Autodesk Fusion 360 part; units mm, degrees
(part 2 of 2)
sketch "Sketch10" plane through (25, 0, 0) normal (-1, 0, 0) x (0, -1, 0)
  arc A0 (-34, 37) -> (-40, 31) centre (-34, 31) ccw
  line L0 (-40, 31) -> (-40, 5)
  line L1 (-40, 5) -> (-10, 5)
  line L2 (-10, 5) -> (-10, 31)
  arc A1 (-10, 31) -> (-16, 37) centre (-16, 31) ccw
  line L3 (-16, 37) -> (-34, 37)
  arc A2 (-21.0078, 28.25) -> (-28.9922, 28.25) centre (-25, 28.5) ccw
  arc A3 (-21.0001, 28.0281) -> (-21.0078, 28.25) centre (-25, 28) ccw
  line L4 (-21.0001, 28.0281) -> (-22.5107, 11.7687)
  arc A4 (-27.4899, 11.7754) -> (-22.5107, 11.7687) centre (-25, 12) ccw
  line L5 (-27.4899, 11.7754) -> (-28.8938, 27.1715)
  line L6 (-28.8938, 27.1715) -> (-28.9999, 28.0281)
  arc A5 (-28.9922, 28.25) -> (-28.9999, 28.0281) centre (-25, 28) ccw
  circle A6 centre (-25, 28.5) radius 4
  circle A7 centre (-25, 12) radius 2.5
  line L7 (-22.5107, 11.7687) -> (-21.0001, 28.0281)
  line L8 (-28.9999, 28.0281) -> (-27.4899, 11.7754)
  constraint concentric A2 A6
  constraint concentric A4 A7
  constraint coincident L4.end A4.end
  constraint coincident A3.start L4.start
  constraint coincident L6.end A5.end
  constraint coincident A4.start L5.start
extrude "Extrude8" add sketch "Sketch10" against normal blind 3 contours A3 L4 L5 L6 A5 A6 A7 L7 | A4 A7
sketch "Sketch11" plane through (0, 0, 0) normal (0, 0, -1) x (1, 0, 0)
  arc A0 (14, 0) -> (0, -14) centre (14, -14) ccw
  line L0 (0, -14) -> (0, -36)
  arc A1 (0, -36) -> (14, -50) centre (14, -36) ccw
  line L1 (14, -50) -> (26, -50)
  arc A2 (26, -50) -> (40, -36) centre (26, -36) ccw
  line L2 (40, -36) -> (40, -14)
  arc A3 (40, -14) -> (26, 0) centre (26, -14) ccw
  line L3 (26, 0) -> (14, 0)
sketch "Sketch12" plane through (0, 0, 0) normal (0, -1, 0) x (1, 0, 0)
  line L0 (14, 5) -> (14, 0)
  line L1 (14, 0) -> (26, 0)
  line L2 (26, 0) -> (26, 5)
  line L3 (26, 5) -> (14, 5)
  line L4 (0, 0) -> (40, 0)
  line L5 (40, 0) -> (40, 2)
  line L6 (40, 2) -> (0, 2)
  line L7 (0, 2) -> (0, 0)
  constraint horizontal L4
  constraint vertical L5
  constraint horizontal L6
  constraint vertical L7
  constraint coincident L4.start L7.end
extrude "Extrude9" cut sketch "Sketch12" against normal blind 50 contours L0 L1 L2 L4 L6 | L0 L4 L6 L7 | L2 L4 L5 L6
sketch "Sketch13" plane through (30, 0, 0) normal (1, 0, 0) x (0, 1, 0)
  arc A0 (28.9922, 28.25) -> (21.0078, 28.25) centre (25, 28.5) ccw
  arc A1 (28.9999, 28.0281) -> (28.9922, 28.25) centre (25, 28) ccw
  line L0 (28.9999, 28.0281) -> (28.8938, 27.1715)
  line L1 (28.8938, 27.1715) -> (27.4899, 11.7754)
  arc A2 (22.5107, 11.7687) -> (27.4899, 11.7754) centre (25, 12) ccw
  line L2 (22.5107, 11.7687) -> (21.0001, 28.0281)
  arc A3 (21.0078, 28.25) -> (21.0001, 28.0281) centre (25, 28) ccw
  arc A4 (40, 31) -> (34, 37) centre (34, 31) ccw
  line L3 (34, 37) -> (16, 37)
  arc A5 (16, 37) -> (10, 31) centre (16, 31) ccw
  line L4 (10, 31) -> (10, 5)
  line L5 (10, 5) -> (40, 5)
  line L6 (40, 5) -> (40, 31)
  line L7 (15, 35) -> (35, 35)
  line L8 (35, 35) -> (35, 5)
  line L9 (35, 5) -> (15, 5)
  line L10 (15, 5) -> (15, 35)
  line L11 (9, 38) -> (41, 38)
  line L12 (41, 38) -> (41, 5)
  line L13 (41, 5) -> (9, 5)
  line L14 (9, 5) -> (9, 38)
  constraint horizontal L7
  constraint vertical L8
  constraint horizontal L9
  constraint vertical L10
  constraint horizontal L11
  constraint vertical L12
  constraint horizontal L13
  constraint vertical L14
extrude "Extrude10" cut sketch "Sketch13" against normal blind 5 contours A4 L3 A5 L4 L5 L6 L7 L8 L10 L13 | A4 L3 A5 L4 L6 L11 L12 L13 L14
sketch "Sketch14" plane through (0, 0, 0) normal (0, 0, -1) x (1, 0, 0)
  line L0 (7, -5) -> (35, -5)
  line L1 (35, -5) -> (35, -45)
  line L2 (35, -45) -> (7, -45)
  line L3 (7, -45) -> (7, -5)
  line L4 (0, 0) -> (40, 0)
  line L5 (40, 0) -> (40, -50)
  line L6 (40, -50) -> (0, -50)
  line L7 (0, -50) -> (0, 0)
  constraint horizontal L0
  constraint vertical L1
  constraint horizontal L2
  constraint vertical L3
  constraint horizontal L4
  constraint vertical L5
  constraint horizontal L6
  constraint vertical L7
  constraint coincident L4.start L7.end
extrude "Extrude11" cut sketch "Sketch14" against normal blind 5
fillet "Fillet3" radius 4.5 4 edges at (7, 45, 3.5) (7, 5, 3.5) (35, 45, 3.5) (35, 5, 3.5)
fillet "Fillet4" radius 7 2 edges at (27.5, 15, 35) (27.5, 35, 35)
